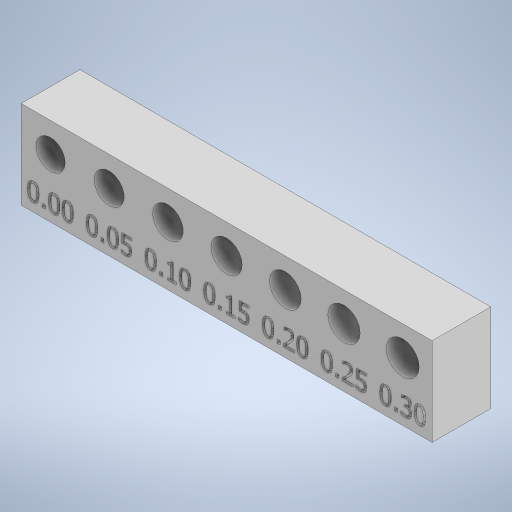
# Autodesk Inventor part: FIT TEST
Saved by Autodesk Inventor 2023 (Build 270158000, 158)
## iProperties
Created: 2023-05-17
Part Number: FIT TEST
Material: Generic
Document SubType Name: Modeling
Designer: Louis
Density: 1 g/cm^3
Appearance: Default
Author: Louis
Autodesk Inventor part; units mm, degrees
ref_plane "YZ Plane" through (0, 0, 0) normal (1, 0, 0) x (0, 1, 0)
ref_plane "XZ Plane" through (0, 0, 0) normal (0, 1, 0) x (-1, 0, 0)
ref_plane "XY Plane" through (0, 0, 0) normal (0, 0, 1) x (1, 0, 0)
sketch "Sketch1" plane through (0, 0, 0) normal (0, 0, 1) x (1, 0, 0)
  line L0 (0, 0) -> (10, 0)
  line L1 (10, 0) -> (10, 15)
  line L2 (10, 15) -> (0, 15)
  line L3 (0, 15) -> (0, 0)
  dimension "d0" = 10
  dimension "d1" = 15
  constraints: 8 end point, 2 parallel, 1 horizontal, 1 perpendicular
  measures "d0" distance of L1.end L2.end
  measures "d1" distance of L0.end L1.end
extrude "Extrusion1" add sketch "Sketch1" along normal blind 10
sketch "Sketch2" plane through (0, 0, 10) normal (0, 0, 1) x (1, 0, 0)
  line L0 (0, 15) -> (0, 0) projected
  line L1 (10, 15) -> (0, 15) projected
  point P0 (5, 10)
  dimension "d4" = 5
  dimension "d12" = 5
  measures "d4" distance from line of L0 point (5, 10)
  measures "d12" distance from line of L1 point (5, 10)
hole "Hole1" at (5, 10, 10) direction (0, 0, -1) diameter 5 end through all
pattern_linear "Rectangular Pattern1" count 7 spacing 10 along (1, 0, 0) of "Hole1", "Extrusion1"
sketch "Sketch3" plane through (0, 0, 10) normal (0, 0, 1) x (1, 0, 0)
  line L0 (0, 15) -> (0, 0) projected
  line L1 (0, 0) -> (10, 0)
  line L2 (10, 0) -> (10, 15)
  line L3 (10, 15) -> (0, 15)
  line L4 (0, 15) -> (0, 0)
  line L5 (10, 0) -> (20, 0)
  line L6 (20, 0) -> (20, 15)
  line L7 (20, 15) -> (10, 15)
  line L8 (10, 15) -> (10, 0)
  line L9 (20, 15) -> (30, 15)
  line L10 (30, 15) -> (30, 0)
  line L11 (30, 0) -> (20, 0)
  line L12 (20, 0) -> (20, 15)
  line L13 (30, 0) -> (40, 0)
  line L14 (40, 0) -> (40, 15)
  line L15 (40, 15) -> (30, 15)
  line L16 (30, 15) -> (30, 0)
  line L17 (40, 15) -> (40, 0)
  line L18 (0.9344, 4.587) -> (9.0656, 4.587) construction
  line L19 (9.0656, 4.587) -> (9.0656, 1.413) construction
  line L20 (9.0656, 1.413) -> (0.9344, 1.413) construction
  line L21 (0.9344, 1.413) -> (0.9344, 4.587) construction
  line L22 (10.9344, 4.587) -> (19.0656, 4.587) construction
  line L23 (19.0656, 4.587) -> (19.0656, 1.413) construction
  line L24 (19.0656, 1.413) -> (10.9344, 1.413) construction
  line L25 (10.9344, 1.413) -> (10.9344, 4.587) construction
  line L26 (20.9344, 4.587) -> (29.0656, 4.587) construction
  line L27 (29.0656, 4.587) -> (29.0656, 1.413) construction
  line L28 (29.0656, 1.413) -> (20.9344, 1.413) construction
  line L29 (20.9344, 1.413) -> (20.9344, 4.587) construction
  line L30 (30.9344, 4.587) -> (39.0656, 4.587) construction
  line L31 (39.0656, 4.587) -> (39.0656, 1.413) construction
  line L32 (39.0656, 1.413) -> (30.9344, 1.413) construction
  line L33 (30.9344, 1.413) -> (30.9344, 4.587) construction
  line L34 (40.9344, 4.5882) -> (49.0656, 4.5882) construction
  line L35 (49.0656, 4.5882) -> (49.0656, 1.4118) construction
  line L36 (49.0656, 1.4118) -> (40.9344, 1.4118) construction
  line L37 (40.9344, 1.4118) -> (40.9344, 4.5882) construction
  line L38 (50.9344, 4.5882) -> (59.0656, 4.5882) construction
  line L39 (59.0656, 4.5882) -> (59.0656, 1.4118) construction
  line L40 (59.0656, 1.4118) -> (50.9344, 1.4118) construction
  line L41 (50.9344, 1.4118) -> (50.9344, 4.5882) construction
  line L42 (60.9344, 4.5882) -> (69.0656, 4.5882) construction
  line L43 (69.0656, 4.5882) -> (69.0656, 1.4118) construction
  line L44 (69.0656, 1.4118) -> (60.9344, 1.4118) construction
  line L45 (60.9344, 1.4118) -> (60.9344, 4.5882) construction
  line L46 (0, 0) -> (70, 0) projected
  line L47 (40, 15) -> (50, 15)
  line L48 (50, 15) -> (50, 0)
  line L49 (50, 0) -> (40, 0)
  line L50 (40, 0) -> (40, 15)
  line L51 (0, 0) -> (70, 0) projected
  line L52 (50, 15) -> (60, 15)
  line L53 (60, 15) -> (60, 0)
  line L54 (60, 0) -> (50, 0)
  line L55 (50, 0) -> (50, 15)
  line L56 (60, 15) -> (70, 15)
  line L57 (70, 15) -> (70, 0)
  line L58 (70, 0) -> (60, 0)
  line L59 (60, 0) -> (60, 15)
  line L60 (70, 0) -> (70, 15) projected
  line L61 (70, 15) -> (0, 15) projected
  line L62 (0, 15) -> (0, 0) projected
  line L63 (0, 3) -> (70, 3)
  spline S0 degree 2 poles (3.0536, 3.0012) (3.0536, 2.1812) (2.5769, 1.413) (2.0804, 1.413) knots 0 0 0 1 2 2 2
  spline S1 degree 2 poles (2.0804, 1.413) (1.5766, 1.413) (1.1048, 2.196) (1.1048, 2.9988) knots 0 0 0 1 2 2 2
  spline S2 degree 2 poles (1.1048, 2.9988) (1.1048, 3.8238) (1.5815, 4.587) (2.0804, 4.587) knots 0 0 0 1 2 2 2
  spline S3 degree 2 poles (2.0804, 4.587) (2.5819, 4.587) (3.0536, 3.7966) (3.0536, 3.0012) knots 0 0 0 1 2 2 2
  spline S4 degree 2 poles (2.53, 2.0725) (2.5893, 2.2232) (2.6387, 2.6875) (2.6387, 3.0012) knots 0 0 0 1 2 2 2
  spline S5 degree 2 poles (2.6387, 3.0012) (2.6387, 3.3149) (2.5893, 3.7768) (2.5275, 3.9324) knots 0 0 0 1 2 2 2
  spline S6 degree 2 poles (2.5275, 3.9324) (2.4658, 4.088) (2.2509, 4.2486) (2.0804, 4.2486) knots 0 0 0 1 2 2 2
  spline S7 degree 2 poles (2.0804, 4.2486) (1.91, 4.2486) (1.6902, 4.088) (1.626, 3.9275) knots 0 0 0 1 2 2 2
  spline S8 degree 2 poles (1.626, 3.9275) (1.5642, 3.7719) (1.5197, 3.2976) (1.5197, 2.9988) knots 0 0 0 1 2 2 2
  spline S9 degree 2 poles (1.5197, 2.9988) (1.5197, 2.6777) (1.5593, 2.2479) (1.6235, 2.0799) knots 0 0 0 1 2 2 2
  spline S10 degree 2 poles (1.6235, 2.0799) (1.6828, 1.9218) (1.9026, 1.7514) (2.0804, 1.7514) knots 0 0 0 1 2 2 2
  spline S11 degree 2 poles (2.0804, 1.7514) (2.2484, 1.7514) (2.4682, 1.912) (2.53, 2.0725) knots 0 0 0 1 2 2 2
  line L64 (4.0984, 1.4772) -> (3.6094, 1.4772)
  line L65 (3.6094, 1.4772) -> (3.6094, 2.0602)
  line L66 (3.6094, 2.0602) -> (4.0984, 2.0602)
  line L67 (4.0984, 2.0602) -> (4.0984, 1.4772)
  spline S12 degree 2 poles (6.6105, 3.0012) (6.6105, 2.1812) (6.1337, 1.413) (5.6373, 1.413) knots 0 0 0 1 2 2 2
  spline S13 degree 2 poles (5.6373, 1.413) (5.1334, 1.413) (4.6616, 2.196) (4.6616, 2.9988) knots 0 0 0 1 2 2 2
  spline S14 degree 2 poles (4.6616, 2.9988) (4.6616, 3.8238) (5.1383, 4.587) (5.6373, 4.587) knots 0 0 0 1 2 2 2
  spline S15 degree 2 poles (5.6373, 4.587) (6.1387, 4.587) (6.6105, 3.7966) (6.6105, 3.0012) knots 0 0 0 1 2 2 2
  spline S16 degree 2 poles (6.0868, 2.0725) (6.1461, 2.2232) (6.1955, 2.6875) (6.1955, 3.0012) knots 0 0 0 1 2 2 2
  spline S17 degree 2 poles (6.1955, 3.0012) (6.1955, 3.3149) (6.1461, 3.7768) (6.0843, 3.9324) knots 0 0 0 1 2 2 2
  spline S18 degree 2 poles (6.0843, 3.9324) (6.0226, 4.088) (5.8077, 4.2486) (5.6373, 4.2486) knots 0 0 0 1 2 2 2
  spline S19 degree 2 poles (5.6373, 4.2486) (5.4668, 4.2486) (5.247, 4.088) (5.1828, 3.9275) knots 0 0 0 1 2 2 2
  spline S20 degree 2 poles (5.1828, 3.9275) (5.121, 3.7719) (5.0766, 3.2976) (5.0766, 2.9988) knots 0 0 0 1 2 2 2
  spline S21 degree 2 poles (5.0766, 2.9988) (5.0766, 2.6777) (5.1161, 2.2479) (5.1803, 2.0799) knots 0 0 0 1 2 2 2
  spline S22 degree 2 poles (5.1803, 2.0799) (5.2396, 1.9218) (5.4594, 1.7514) (5.6373, 1.7514) knots 0 0 0 1 2 2 2
  spline S23 degree 2 poles (5.6373, 1.7514) (5.8052, 1.7514) (6.0251, 1.912) (6.0868, 2.0725) knots 0 0 0 1 2 2 2
  spline S24 degree 2 poles (8.8977, 3.0012) (8.8977, 2.1812) (8.421, 1.413) (7.9245, 1.413) knots 0 0 0 1 2 2 2
  spline S25 degree 2 poles (7.9245, 1.413) (7.4206, 1.413) (6.9488, 2.196) (6.9488, 2.9988) knots 0 0 0 1 2 2 2
  spline S26 degree 2 poles (6.9488, 2.9988) (6.9488, 3.8238) (7.4256, 4.587) (7.9245, 4.587) knots 0 0 0 1 2 2 2
  spline S27 degree 2 poles (7.9245, 4.587) (8.4259, 4.587) (8.8977, 3.7966) (8.8977, 3.0012) knots 0 0 0 1 2 2 2
  spline S28 degree 2 poles (8.374, 2.0725) (8.4333, 2.2232) (8.4827, 2.6875) (8.4827, 3.0012) knots 0 0 0 1 2 2 2
  spline S29 degree 2 poles (8.4827, 3.0012) (8.4827, 3.3149) (8.4333, 3.7768) (8.3716, 3.9324) knots 0 0 0 1 2 2 2
  spline S30 degree 2 poles (8.3716, 3.9324) (8.3098, 4.088) (8.0949, 4.2486) (7.9245, 4.2486) knots 0 0 0 1 2 2 2
  spline S31 degree 2 poles (7.9245, 4.2486) (7.7541, 4.2486) (7.5342, 4.088) (7.47, 3.9275) knots 0 0 0 1 2 2 2
  spline S32 degree 2 poles (7.47, 3.9275) (7.4083, 3.7719) (7.3638, 3.2976) (7.3638, 2.9988) knots 0 0 0 1 2 2 2
  spline S33 degree 2 poles (7.3638, 2.9988) (7.3638, 2.6777) (7.4033, 2.2479) (7.4675, 2.0799) knots 0 0 0 1 2 2 2
  spline S34 degree 2 poles (7.4675, 2.0799) (7.5268, 1.9218) (7.7467, 1.7514) (7.9245, 1.7514) knots 0 0 0 1 2 2 2
  spline S35 degree 2 poles (7.9245, 1.7514) (8.0925, 1.7514) (8.3123, 1.912) (8.374, 2.0725) knots 0 0 0 1 2 2 2
  spline S36 degree 2 poles (13.0536, 3.0012) (13.0536, 2.1812) (12.5769, 1.413) (12.0804, 1.413) knots 0 0 0 1 2 2 2
  spline S37 degree 2 poles (12.0804, 1.413) (11.5766, 1.413) (11.1048, 2.196) (11.1048, 2.9988) knots 0 0 0 1 2 2 2
  spline S38 degree 2 poles (11.1048, 2.9988) (11.1048, 3.8238) (11.5815, 4.587) (12.0804, 4.587) knots 0 0 0 1 2 2 2
  spline S39 degree 2 poles (12.0804, 4.587) (12.5819, 4.587) (13.0536, 3.7966) (13.0536, 3.0012) knots 0 0 0 1 2 2 2
  spline S40 degree 2 poles (12.53, 2.0725) (12.5893, 2.2232) (12.6387, 2.6875) (12.6387, 3.0012) knots 0 0 0 1 2 2 2
  spline S41 degree 2 poles (12.6387, 3.0012) (12.6387, 3.3149) (12.5893, 3.7768) (12.5275, 3.9324) knots 0 0 0 1 2 2 2
  spline S42 degree 2 poles (12.5275, 3.9324) (12.4658, 4.088) (12.2509, 4.2486) (12.0804, 4.2486) knots 0 0 0 1 2 2 2
  spline S43 degree 2 poles (12.0804, 4.2486) (11.91, 4.2486) (11.6902, 4.088) (11.626, 3.9275) knots 0 0 0 1 2 2 2
  spline S44 degree 2 poles (11.626, 3.9275) (11.5642, 3.7719) (11.5197, 3.2976) (11.5197, 2.9988) knots 0 0 0 1 2 2 2
  spline S45 degree 2 poles (11.5197, 2.9988) (11.5197, 2.6777) (11.5593, 2.2479) (11.6235, 2.0799) knots 0 0 0 1 2 2 2
  spline S46 degree 2 poles (11.6235, 2.0799) (11.6828, 1.9218) (11.9026, 1.7514) (12.0804, 1.7514) knots 0 0 0 1 2 2 2
  spline S47 degree 2 poles (12.0804, 1.7514) (12.2484, 1.7514) (12.4682, 1.912) (12.53, 2.0725) knots 0 0 0 1 2 2 2
  line L68 (14.0984, 1.4772) -> (13.6094, 1.4772)
  line L69 (13.6094, 1.4772) -> (13.6094, 2.0602)
  line L70 (13.6094, 2.0602) -> (14.0984, 2.0602)
  line L71 (14.0984, 2.0602) -> (14.0984, 1.4772)
  spline S48 degree 2 poles (16.6105, 3.0012) (16.6105, 2.1812) (16.1337, 1.413) (15.6373, 1.413) knots 0 0 0 1 2 2 2
  spline S49 degree 2 poles (15.6373, 1.413) (15.1334, 1.413) (14.6616, 2.196) (14.6616, 2.9988) knots 0 0 0 1 2 2 2
  spline S50 degree 2 poles (14.6616, 2.9988) (14.6616, 3.8238) (15.1383, 4.587) (15.6373, 4.587) knots 0 0 0 1 2 2 2
  spline S51 degree 2 poles (15.6373, 4.587) (16.1387, 4.587) (16.6105, 3.7966) (16.6105, 3.0012) knots 0 0 0 1 2 2 2
  spline S52 degree 2 poles (16.0868, 2.0725) (16.1461, 2.2232) (16.1955, 2.6875) (16.1955, 3.0012) knots 0 0 0 1 2 2 2
  spline S53 degree 2 poles (16.1955, 3.0012) (16.1955, 3.3149) (16.1461, 3.7768) (16.0843, 3.9324) knots 0 0 0 1 2 2 2
  spline S54 degree 2 poles (16.0843, 3.9324) (16.0226, 4.088) (15.8077, 4.2486) (15.6373, 4.2486) knots 0 0 0 1 2 2 2
  spline S55 degree 2 poles (15.6373, 4.2486) (15.4668, 4.2486) (15.247, 4.088) (15.1828, 3.9275) knots 0 0 0 1 2 2 2
  spline S56 degree 2 poles (15.1828, 3.9275) (15.121, 3.7719) (15.0766, 3.2976) (15.0766, 2.9988) knots 0 0 0 1 2 2 2
  spline S57 degree 2 poles (15.0766, 2.9988) (15.0766, 2.6777) (15.1161, 2.2479) (15.1803, 2.0799) knots 0 0 0 1 2 2 2
  spline S58 degree 2 poles (15.1803, 2.0799) (15.2396, 1.9218) (15.4594, 1.7514) (15.6373, 1.7514) knots 0 0 0 1 2 2 2
  spline S59 degree 2 poles (15.6373, 1.7514) (15.8052, 1.7514) (16.0251, 1.912) (16.0868, 2.0725) knots 0 0 0 1 2 2 2
  spline S60 degree 2 poles (18.8483, 2.4455) (18.8483, 2.2256) (18.7075, 1.8502) (18.5791, 1.7119) knots 0 0 0 1 2 2 2
  spline S61 degree 2 poles (18.5791, 1.7119) (18.4506, 1.5736) (18.0678, 1.413) (17.8306, 1.413) knots 0 0 0 1 2 2 2
  spline S62 degree 2 poles (17.8306, 1.413) (17.6133, 1.413) (17.1884, 1.5093) (17.0328, 1.5859) knots 0 0 0 1 2 2 2
  line L72 (17.0328, 1.5859) -> (17.0328, 2.0182)
  line L73 (17.0328, 2.0182) -> (17.0625, 2.0182)
  spline S63 degree 2 poles (17.0625, 2.0182) (17.1094, 1.9836) (17.2848, 1.8947) (17.391, 1.8551) knots 0 0 0 1 2 2 2
  spline S64 degree 2 poles (17.391, 1.8551) (17.512, 1.8132) (17.7121, 1.7662) (17.838, 1.7662) knots 0 0 0 1 2 2 2
  spline S65 degree 2 poles (17.838, 1.7662) (17.9615, 1.7662) (18.1937, 1.8551) (18.2777, 1.9515) knots 0 0 0 1 2 2 2
  spline S66 degree 2 poles (18.2777, 1.9515) (18.3543, 2.0429) (18.4333, 2.2849) (18.4333, 2.448) knots 0 0 0 1 2 2 2
  spline S67 degree 2 poles (18.4333, 2.448) (18.4333, 2.611) (18.3444, 2.8185) (18.2604, 2.8876) knots 0 0 0 1 2 2 2
  spline S68 degree 2 poles (18.2604, 2.8876) (18.174, 2.9642) (17.9171, 3.0284) (17.7615, 3.0284) knots 0 0 0 1 2 2 2
  spline S69 degree 2 poles (17.7615, 3.0284) (17.5935, 3.0284) (17.2601, 2.9765) (17.1588, 2.9543) knots 0 0 0 1 2 2 2
  line L74 (17.1588, 2.9543) -> (17.1588, 4.5252)
  line L75 (17.1588, 4.5252) -> (18.831, 4.5252)
  line L76 (18.831, 4.5252) -> (18.831, 4.1671)
  line L77 (18.831, 4.1671) -> (17.5515, 4.1671)
  line L78 (17.5515, 4.1671) -> (17.5515, 3.3544)
  spline S70 degree 2 poles (17.5515, 3.3544) (17.6256, 3.3643) (17.7689, 3.3717) (17.8282, 3.3717) knots 0 0 0 1 2 2 2
  spline S71 degree 2 poles (17.8282, 3.3717) (18.0628, 3.3717) (18.3864, 3.2952) (18.5346, 3.1815) knots 0 0 0 1 2 2 2
  spline S72 degree 2 poles (18.5346, 3.1815) (18.6853, 3.0679) (18.8483, 2.7221) (18.8483, 2.4455) knots 0 0 0 1 2 2 2
  spline S73 degree 2 poles (23.0536, 3.0012) (23.0536, 2.1812) (22.5769, 1.413) (22.0804, 1.413) knots 0 0 0 1 2 2 2
  spline S74 degree 2 poles (22.0804, 1.413) (21.5766, 1.413) (21.1048, 2.196) (21.1048, 2.9988) knots 0 0 0 1 2 2 2
  spline S75 degree 2 poles (21.1048, 2.9988) (21.1048, 3.8238) (21.5815, 4.587) (22.0804, 4.587) knots 0 0 0 1 2 2 2
  spline S76 degree 2 poles (22.0804, 4.587) (22.5819, 4.587) (23.0536, 3.7966) (23.0536, 3.0012) knots 0 0 0 1 2 2 2
  spline S77 degree 2 poles (22.53, 2.0725) (22.5893, 2.2232) (22.6387, 2.6875) (22.6387, 3.0012) knots 0 0 0 1 2 2 2
  spline S78 degree 2 poles (22.6387, 3.0012) (22.6387, 3.3149) (22.5893, 3.7768) (22.5275, 3.9324) knots 0 0 0 1 2 2 2
  spline S79 degree 2 poles (22.5275, 3.9324) (22.4658, 4.088) (22.2509, 4.2486) (22.0804, 4.2486) knots 0 0 0 1 2 2 2
  spline S80 degree 2 poles (22.0804, 4.2486) (21.91, 4.2486) (21.6902, 4.088) (21.626, 3.9275) knots 0 0 0 1 2 2 2
  spline S81 degree 2 poles (21.626, 3.9275) (21.5642, 3.7719) (21.5197, 3.2976) (21.5197, 2.9988) knots 0 0 0 1 2 2 2
  spline S82 degree 2 poles (21.5197, 2.9988) (21.5197, 2.6777) (21.5593, 2.2479) (21.6235, 2.0799) knots 0 0 0 1 2 2 2
  spline S83 degree 2 poles (21.6235, 2.0799) (21.6828, 1.9218) (21.9026, 1.7514) (22.0804, 1.7514) knots 0 0 0 1 2 2 2
  spline S84 degree 2 poles (22.0804, 1.7514) (22.2484, 1.7514) (22.4682, 1.912) (22.53, 2.0725) knots 0 0 0 1 2 2 2
  line L79 (24.0984, 1.4772) -> (23.6094, 1.4772)
  line L80 (23.6094, 1.4772) -> (23.6094, 2.0602)
  line L81 (23.6094, 2.0602) -> (24.0984, 2.0602)
  line L82 (24.0984, 2.0602) -> (24.0984, 1.4772)
  line L83 (26.44, 1.4772) -> (24.9531, 1.4772)
  line L84 (24.9531, 1.4772) -> (24.9531, 1.7885)
  line L85 (24.9531, 1.7885) -> (25.5064, 1.7885)
  line L86 (25.5064, 1.7885) -> (25.5064, 3.8312)
  line L87 (25.5064, 3.8312) -> (24.9531, 3.8312)
  line L88 (24.9531, 3.8312) -> (24.9531, 4.1103)
  spline S85 degree 2 poles (24.9531, 4.1103) (25.2668, 4.1103) (25.5632, 4.2881) (25.5829, 4.5351) knots 0 0 0 1 2 2 2
  line L89 (25.5829, 4.5351) -> (25.8991, 4.5351)
  line L90 (25.8991, 4.5351) -> (25.8991, 1.7885)
  line L91 (25.8991, 1.7885) -> (26.44, 1.7885)
  line L92 (26.44, 1.7885) -> (26.44, 1.4772)
  spline S86 degree 2 poles (28.8977, 3.0012) (28.8977, 2.1812) (28.421, 1.413) (27.9245, 1.413) knots 0 0 0 1 2 2 2
  spline S87 degree 2 poles (27.9245, 1.413) (27.4206, 1.413) (26.9488, 2.196) (26.9488, 2.9988) knots 0 0 0 1 2 2 2
  spline S88 degree 2 poles (26.9488, 2.9988) (26.9488, 3.8238) (27.4256, 4.587) (27.9245, 4.587) knots 0 0 0 1 2 2 2
  spline S89 degree 2 poles (27.9245, 4.587) (28.4259, 4.587) (28.8977, 3.7966) (28.8977, 3.0012) knots 0 0 0 1 2 2 2
  spline S90 degree 2 poles (28.374, 2.0725) (28.4333, 2.2232) (28.4827, 2.6875) (28.4827, 3.0012) knots 0 0 0 1 2 2 2
  spline S91 degree 2 poles (28.4827, 3.0012) (28.4827, 3.3149) (28.4333, 3.7768) (28.3716, 3.9324) knots 0 0 0 1 2 2 2
  spline S92 degree 2 poles (28.3716, 3.9324) (28.3098, 4.088) (28.0949, 4.2486) (27.9245, 4.2486) knots 0 0 0 1 2 2 2
  spline S93 degree 2 poles (27.9245, 4.2486) (27.7541, 4.2486) (27.5342, 4.088) (27.47, 3.9275) knots 0 0 0 1 2 2 2
  spline S94 degree 2 poles (27.47, 3.9275) (27.4083, 3.7719) (27.3638, 3.2976) (27.3638, 2.9988) knots 0 0 0 1 2 2 2
  spline S95 degree 2 poles (27.3638, 2.9988) (27.3638, 2.6777) (27.4033, 2.2479) (27.4675, 2.0799) knots 0 0 0 1 2 2 2
  spline S96 degree 2 poles (27.4675, 2.0799) (27.5268, 1.9218) (27.7467, 1.7514) (27.9245, 1.7514) knots 0 0 0 1 2 2 2
  spline S97 degree 2 poles (27.9245, 1.7514) (28.0925, 1.7514) (28.3123, 1.912) (28.374, 2.0725) knots 0 0 0 1 2 2 2
  spline S98 degree 2 poles (33.0536, 3.0012) (33.0536, 2.1812) (32.5769, 1.413) (32.0804, 1.413) knots 0 0 0 1 2 2 2
  spline S99 degree 2 poles (32.0804, 1.413) (31.5766, 1.413) (31.1048, 2.196) (31.1048, 2.9988) knots 0 0 0 1 2 2 2
  spline S100 degree 2 poles (31.1048, 2.9988) (31.1048, 3.8238) (31.5815, 4.587) (32.0804, 4.587) knots 0 0 0 1 2 2 2
  spline S101 degree 2 poles (32.0804, 4.587) (32.5819, 4.587) (33.0536, 3.7966) (33.0536, 3.0012) knots 0 0 0 1 2 2 2
  spline S102 degree 2 poles (32.53, 2.0725) (32.5893, 2.2232) (32.6387, 2.6875) (32.6387, 3.0012) knots 0 0 0 1 2 2 2
  spline S103 degree 2 poles (32.6387, 3.0012) (32.6387, 3.3149) (32.5893, 3.7768) (32.5275, 3.9324) knots 0 0 0 1 2 2 2
  spline S104 degree 2 poles (32.5275, 3.9324) (32.4658, 4.088) (32.2509, 4.2486) (32.0804, 4.2486) knots 0 0 0 1 2 2 2
  spline S105 degree 2 poles (32.0804, 4.2486) (31.91, 4.2486) (31.6902, 4.088) (31.626, 3.9275) knots 0 0 0 1 2 2 2
  spline S106 degree 2 poles (31.626, 3.9275) (31.5642, 3.7719) (31.5197, 3.2976) (31.5197, 2.9988) knots 0 0 0 1 2 2 2
  spline S107 degree 2 poles (31.5197, 2.9988) (31.5197, 2.6777) (31.5593, 2.2479) (31.6235, 2.0799) knots 0 0 0 1 2 2 2
  spline S108 degree 2 poles (31.6235, 2.0799) (31.6828, 1.9218) (31.9026, 1.7514) (32.0804, 1.7514) knots 0 0 0 1 2 2 2
  spline S109 degree 2 poles (32.0804, 1.7514) (32.2484, 1.7514) (32.4682, 1.912) (32.53, 2.0725) knots 0 0 0 1 2 2 2
  line L93 (34.0984, 1.4772) -> (33.6094, 1.4772)
  line L94 (33.6094, 1.4772) -> (33.6094, 2.0602)
  line L95 (33.6094, 2.0602) -> (34.0984, 2.0602)
  line L96 (34.0984, 2.0602) -> (34.0984, 1.4772)
  line L97 (36.44, 1.4772) -> (34.9531, 1.4772)
  line L98 (34.9531, 1.4772) -> (34.9531, 1.7885)
  line L99 (34.9531, 1.7885) -> (35.5064, 1.7885)
  line L100 (35.5064, 1.7885) -> (35.5064, 3.8312)
  line L101 (35.5064, 3.8312) -> (34.9531, 3.8312)
  line L102 (34.9531, 3.8312) -> (34.9531, 4.1103)
  spline S110 degree 2 poles (34.9531, 4.1103) (35.2668, 4.1103) (35.5632, 4.2881) (35.5829, 4.5351) knots 0 0 0 1 2 2 2
  line L103 (35.5829, 4.5351) -> (35.8991, 4.5351)
  line L104 (35.8991, 4.5351) -> (35.8991, 1.7885)
  line L105 (35.8991, 1.7885) -> (36.44, 1.7885)
  line L106 (36.44, 1.7885) -> (36.44, 1.4772)
  spline S111 degree 2 poles (38.8483, 2.4455) (38.8483, 2.2256) (38.7075, 1.8502) (38.5791, 1.7119) knots 0 0 0 1 2 2 2
  spline S112 degree 2 poles (38.5791, 1.7119) (38.4506, 1.5736) (38.0678, 1.413) (37.8306, 1.413) knots 0 0 0 1 2 2 2
  spline S113 degree 2 poles (37.8306, 1.413) (37.6133, 1.413) (37.1884, 1.5093) (37.0328, 1.5859) knots 0 0 0 1 2 2 2
  line L107 (37.0328, 1.5859) -> (37.0328, 2.0182)
  line L108 (37.0328, 2.0182) -> (37.0625, 2.0182)
  spline S114 degree 2 poles (37.0625, 2.0182) (37.1094, 1.9836) (37.2848, 1.8947) (37.391, 1.8551) knots 0 0 0 1 2 2 2
  spline S115 degree 2 poles (37.391, 1.8551) (37.512, 1.8132) (37.7121, 1.7662) (37.838, 1.7662) knots 0 0 0 1 2 2 2
  spline S116 degree 2 poles (37.838, 1.7662) (37.9615, 1.7662) (38.1937, 1.8551) (38.2777, 1.9515) knots 0 0 0 1 2 2 2
  spline S117 degree 2 poles (38.2777, 1.9515) (38.3543, 2.0429) (38.4333, 2.2849) (38.4333, 2.448) knots 0 0 0 1 2 2 2
  spline S118 degree 2 poles (38.4333, 2.448) (38.4333, 2.611) (38.3444, 2.8185) (38.2604, 2.8876) knots 0 0 0 1 2 2 2
  spline S119 degree 2 poles (38.2604, 2.8876) (38.174, 2.9642) (37.9171, 3.0284) (37.7615, 3.0284) knots 0 0 0 1 2 2 2
  spline S120 degree 2 poles (37.7615, 3.0284) (37.5935, 3.0284) (37.2601, 2.9765) (37.1588, 2.9543) knots 0 0 0 1 2 2 2
  line L109 (37.1588, 2.9543) -> (37.1588, 4.5252)
  line L110 (37.1588, 4.5252) -> (38.831, 4.5252)
  line L111 (38.831, 4.5252) -> (38.831, 4.1671)
  line L112 (38.831, 4.1671) -> (37.5515, 4.1671)
  line L113 (37.5515, 4.1671) -> (37.5515, 3.3544)
  spline S121 degree 2 poles (37.5515, 3.3544) (37.6256, 3.3643) (37.7689, 3.3717) (37.8282, 3.3717) knots 0 0 0 1 2 2 2
  spline S122 degree 2 poles (37.8282, 3.3717) (38.0628, 3.3717) (38.3864, 3.2952) (38.5346, 3.1815) knots 0 0 0 1 2 2 2
  spline S123 degree 2 poles (38.5346, 3.1815) (38.6853, 3.0679) (38.8483, 2.7221) (38.8483, 2.4455) knots 0 0 0 1 2 2 2
  spline S124 degree 2 poles (43.0536, 3) (43.0536, 2.18) (42.5769, 1.4118) (42.0804, 1.4118) knots 0 0 0 1 2 2 2
  spline S125 degree 2 poles (42.0804, 1.4118) (41.5766, 1.4118) (41.1048, 2.1948) (41.1048, 2.9975) knots 0 0 0 1 2 2 2
  spline S126 degree 2 poles (41.1048, 2.9975) (41.1048, 3.8225) (41.5815, 4.5858) (42.0804, 4.5858) knots 0 0 0 1 2 2 2
  spline S127 degree 2 poles (42.0804, 4.5858) (42.5819, 4.5858) (43.0536, 3.7953) (43.0536, 3) knots 0 0 0 1 2 2 2
  spline S128 degree 2 poles (42.53, 2.0713) (42.5893, 2.2219) (42.6387, 2.6863) (42.6387, 3) knots 0 0 0 1 2 2 2
  spline S129 degree 2 poles (42.6387, 3) (42.6387, 3.3137) (42.5893, 3.7756) (42.5275, 3.9312) knots 0 0 0 1 2 2 2
  spline S130 degree 2 poles (42.5275, 3.9312) (42.4658, 4.0868) (42.2509, 4.2474) (42.0804, 4.2474) knots 0 0 0 1 2 2 2
  spline S131 degree 2 poles (42.0804, 4.2474) (41.91, 4.2474) (41.6902, 4.0868) (41.626, 3.9263) knots 0 0 0 1 2 2 2
  spline S132 degree 2 poles (41.626, 3.9263) (41.5642, 3.7706) (41.5197, 3.2964) (41.5197, 2.9975) knots 0 0 0 1 2 2 2
  spline S133 degree 2 poles (41.5197, 2.9975) (41.5197, 2.6764) (41.5593, 2.2466) (41.6235, 2.0787) knots 0 0 0 1 2 2 2
  spline S134 degree 2 poles (41.6235, 2.0787) (41.6828, 1.9206) (41.9026, 1.7502) (42.0804, 1.7502) knots 0 0 0 1 2 2 2
  spline S135 degree 2 poles (42.0804, 1.7502) (42.2484, 1.7502) (42.4682, 1.9107) (42.53, 2.0713) knots 0 0 0 1 2 2 2
  line L114 (44.0984, 1.476) -> (43.6094, 1.476)
  line L115 (43.6094, 1.476) -> (43.6094, 2.0589)
  line L116 (43.6094, 2.0589) -> (44.0984, 2.0589)
  line L117 (44.0984, 2.0589) -> (44.0984, 1.476)
  line L118 (46.5932, 1.476) -> (44.7135, 1.476)
  line L119 (44.7135, 1.476) -> (44.7135, 1.9083)
  spline S136 degree 2 poles (44.7135, 1.9083) (44.916, 2.0984) (45.2766, 2.4517) (45.4495, 2.6418) knots 0 0 0 1 2 2 2
  spline S137 degree 2 poles (45.4495, 2.6418) (45.7978, 3.0247) (46.0522, 3.4841) (46.0522, 3.7287) knots 0 0 0 1 2 2 2
  spline S138 degree 2 poles (46.0522, 3.7287) (46.0522, 3.8571) (45.9732, 4.0498) (45.9016, 4.1115) knots 0 0 0 1 2 2 2
  spline S139 degree 2 poles (45.9016, 4.1115) (45.8299, 4.1733) (45.6422, 4.235) (45.5286, 4.235) knots 0 0 0 1 2 2 2
  spline S140 degree 2 poles (45.5286, 4.235) (45.4199, 4.235) (45.1976, 4.1807) (45.0963, 4.1387) knots 0 0 0 1 2 2 2
  spline S141 degree 2 poles (45.0963, 4.1387) (45.0099, 4.1041) (44.8493, 4.0053) (44.7999, 3.9707) knots 0 0 0 1 2 2 2
  line L120 (44.7999, 3.9707) -> (44.7777, 3.9707)
  line L121 (44.7777, 3.9707) -> (44.7777, 4.4054)
  spline S142 degree 2 poles (44.7777, 4.4054) (44.9037, 4.4672) (45.3557, 4.5882) (45.5582, 4.5882) knots 0 0 0 1 2 2 2
  spline S143 degree 2 poles (45.5582, 4.5882) (45.9855, 4.5882) (46.4672, 4.1362) (46.4672, 3.7509) knots 0 0 0 1 2 2 2
  spline S144 degree 2 poles (46.4672, 3.7509) (46.4672, 3.5706) (46.3832, 3.2692) (46.3091, 3.1408) knots 0 0 0 1 2 2 2
  spline S145 degree 2 poles (46.3091, 3.1408) (46.235, 3.0074) (46.0201, 2.7456) (45.9016, 2.6196) knots 0 0 0 1 2 2 2
  spline S146 degree 2 poles (45.9016, 2.6196) (45.7089, 2.4097) (45.2371, 1.9601) (45.0963, 1.8292) knots 0 0 0 1 2 2 2
  line L122 (45.0963, 1.8292) -> (46.5932, 1.8292)
  line L123 (46.5932, 1.8292) -> (46.5932, 1.476)
  spline S147 degree 2 poles (48.8977, 3) (48.8977, 2.18) (48.421, 1.4118) (47.9245, 1.4118) knots 0 0 0 1 2 2 2
  spline S148 degree 2 poles (47.9245, 1.4118) (47.4206, 1.4118) (46.9488, 2.1948) (46.9488, 2.9975) knots 0 0 0 1 2 2 2
  spline S149 degree 2 poles (46.9488, 2.9975) (46.9488, 3.8225) (47.4256, 4.5858) (47.9245, 4.5858) knots 0 0 0 1 2 2 2
  spline S150 degree 2 poles (47.9245, 4.5858) (48.4259, 4.5858) (48.8977, 3.7953) (48.8977, 3) knots 0 0 0 1 2 2 2
  spline S151 degree 2 poles (48.374, 2.0713) (48.4333, 2.2219) (48.4827, 2.6863) (48.4827, 3) knots 0 0 0 1 2 2 2
  spline S152 degree 2 poles (48.4827, 3) (48.4827, 3.3137) (48.4333, 3.7756) (48.3716, 3.9312) knots 0 0 0 1 2 2 2
  spline S153 degree 2 poles (48.3716, 3.9312) (48.3098, 4.0868) (48.0949, 4.2474) (47.9245, 4.2474) knots 0 0 0 1 2 2 2
  spline S154 degree 2 poles (47.9245, 4.2474) (47.7541, 4.2474) (47.5342, 4.0868) (47.47, 3.9263) knots 0 0 0 1 2 2 2
  spline S155 degree 2 poles (47.47, 3.9263) (47.4083, 3.7706) (47.3638, 3.2964) (47.3638, 2.9975) knots 0 0 0 1 2 2 2
  spline S156 degree 2 poles (47.3638, 2.9975) (47.3638, 2.6764) (47.4033, 2.2466) (47.4675, 2.0787) knots 0 0 0 1 2 2 2
  spline S157 degree 2 poles (47.4675, 2.0787) (47.5268, 1.9206) (47.7467, 1.7502) (47.9245, 1.7502) knots 0 0 0 1 2 2 2
  spline S158 degree 2 poles (47.9245, 1.7502) (48.0925, 1.7502) (48.3123, 1.9107) (48.374, 2.0713) knots 0 0 0 1 2 2 2
  spline S159 degree 2 poles (53.0536, 3) (53.0536, 2.18) (52.5769, 1.4118) (52.0804, 1.4118) knots 0 0 0 1 2 2 2
  spline S160 degree 2 poles (52.0804, 1.4118) (51.5766, 1.4118) (51.1048, 2.1948) (51.1048, 2.9975) knots 0 0 0 1 2 2 2
  spline S161 degree 2 poles (51.1048, 2.9975) (51.1048, 3.8225) (51.5815, 4.5858) (52.0804, 4.5858) knots 0 0 0 1 2 2 2
  spline S162 degree 2 poles (52.0804, 4.5858) (52.5819, 4.5858) (53.0536, 3.7953) (53.0536, 3) knots 0 0 0 1 2 2 2
  spline S163 degree 2 poles (52.53, 2.0713) (52.5893, 2.2219) (52.6387, 2.6863) (52.6387, 3) knots 0 0 0 1 2 2 2
  spline S164 degree 2 poles (52.6387, 3) (52.6387, 3.3137) (52.5893, 3.7756) (52.5275, 3.9312) knots 0 0 0 1 2 2 2
  spline S165 degree 2 poles (52.5275, 3.9312) (52.4658, 4.0868) (52.2509, 4.2474) (52.0804, 4.2474) knots 0 0 0 1 2 2 2
  spline S166 degree 2 poles (52.0804, 4.2474) (51.91, 4.2474) (51.6902, 4.0868) (51.626, 3.9263) knots 0 0 0 1 2 2 2
  spline S167 degree 2 poles (51.626, 3.9263) (51.5642, 3.7706) (51.5197, 3.2964) (51.5197, 2.9975) knots 0 0 0 1 2 2 2
  spline S168 degree 2 poles (51.5197, 2.9975) (51.5197, 2.6764) (51.5593, 2.2466) (51.6235, 2.0787) knots 0 0 0 1 2 2 2
  spline S169 degree 2 poles (51.6235, 2.0787) (51.6828, 1.9206) (51.9026, 1.7502) (52.0804, 1.7502) knots 0 0 0 1 2 2 2
  spline S170 degree 2 poles (52.0804, 1.7502) (52.2484, 1.7502) (52.4682, 1.9107) (52.53, 2.0713) knots 0 0 0 1 2 2 2
  line L124 (54.0984, 1.476) -> (53.6094, 1.476)
  line L125 (53.6094, 1.476) -> (53.6094, 2.0589)
  line L126 (53.6094, 2.0589) -> (54.0984, 2.0589)
  line L127 (54.0984, 2.0589) -> (54.0984, 1.476)
  line L128 (56.5932, 1.476) -> (54.7135, 1.476)
  line L129 (54.7135, 1.476) -> (54.7135, 1.9083)
  spline S171 degree 2 poles (54.7135, 1.9083) (54.916, 2.0984) (55.2766, 2.4517) (55.4495, 2.6418) knots 0 0 0 1 2 2 2
  spline S172 degree 2 poles (55.4495, 2.6418) (55.7978, 3.0247) (56.0522, 3.4841) (56.0522, 3.7287) knots 0 0 0 1 2 2 2
  spline S173 degree 2 poles (56.0522, 3.7287) (56.0522, 3.8571) (55.9732, 4.0498) (55.9016, 4.1115) knots 0 0 0 1 2 2 2
  spline S174 degree 2 poles (55.9016, 4.1115) (55.8299, 4.1733) (55.6422, 4.235) (55.5286, 4.235) knots 0 0 0 1 2 2 2
  spline S175 degree 2 poles (55.5286, 4.235) (55.4199, 4.235) (55.1976, 4.1807) (55.0963, 4.1387) knots 0 0 0 1 2 2 2
  spline S176 degree 2 poles (55.0963, 4.1387) (55.0099, 4.1041) (54.8493, 4.0053) (54.7999, 3.9707) knots 0 0 0 1 2 2 2
  line L130 (54.7999, 3.9707) -> (54.7777, 3.9707)
  line L131 (54.7777, 3.9707) -> (54.7777, 4.4054)
  spline S177 degree 2 poles (54.7777, 4.4054) (54.9037, 4.4672) (55.3557, 4.5882) (55.5582, 4.5882) knots 0 0 0 1 2 2 2
  spline S178 degree 2 poles (55.5582, 4.5882) (55.9855, 4.5882) (56.4672, 4.1362) (56.4672, 3.7509) knots 0 0 0 1 2 2 2
  spline S179 degree 2 poles (56.4672, 3.7509) (56.4672, 3.5706) (56.3832, 3.2692) (56.3091, 3.1408) knots 0 0 0 1 2 2 2
  spline S180 degree 2 poles (56.3091, 3.1408) (56.235, 3.0074) (56.0201, 2.7456) (55.9016, 2.6196) knots 0 0 0 1 2 2 2
  spline S181 degree 2 poles (55.9016, 2.6196) (55.7089, 2.4097) (55.2371, 1.9601) (55.0963, 1.8292) knots 0 0 0 1 2 2 2
  line L132 (55.0963, 1.8292) -> (56.5932, 1.8292)
  line L133 (56.5932, 1.8292) -> (56.5932, 1.476)
  spline S182 degree 2 poles (58.8483, 2.4442) (58.8483, 2.2244) (58.7075, 1.849) (58.5791, 1.7107) knots 0 0 0 1 2 2 2
  spline S183 degree 2 poles (58.5791, 1.7107) (58.4506, 1.5723) (58.0678, 1.4118) (57.8306, 1.4118) knots 0 0 0 1 2 2 2
  spline S184 degree 2 poles (57.8306, 1.4118) (57.6133, 1.4118) (57.1884, 1.5081) (57.0328, 1.5847) knots 0 0 0 1 2 2 2
  line L134 (57.0328, 1.5847) -> (57.0328, 2.0169)
  line L135 (57.0328, 2.0169) -> (57.0625, 2.0169)
  spline S185 degree 2 poles (57.0625, 2.0169) (57.1094, 1.9824) (57.2848, 1.8934) (57.391, 1.8539) knots 0 0 0 1 2 2 2
  spline S186 degree 2 poles (57.391, 1.8539) (57.512, 1.8119) (57.7121, 1.765) (57.838, 1.765) knots 0 0 0 1 2 2 2
  spline S187 degree 2 poles (57.838, 1.765) (57.9615, 1.765) (58.1937, 1.8539) (58.2777, 1.9502) knots 0 0 0 1 2 2 2
  spline S188 degree 2 poles (58.2777, 1.9502) (58.3543, 2.0416) (58.4333, 2.2837) (58.4333, 2.4467) knots 0 0 0 1 2 2 2
  spline S189 degree 2 poles (58.4333, 2.4467) (58.4333, 2.6097) (58.3444, 2.8172) (58.2604, 2.8864) knots 0 0 0 1 2 2 2
  spline S190 degree 2 poles (58.2604, 2.8864) (58.174, 2.9629) (57.9171, 3.0272) (57.7615, 3.0272) knots 0 0 0 1 2 2 2
  spline S191 degree 2 poles (57.7615, 3.0272) (57.5935, 3.0272) (57.2601, 2.9753) (57.1588, 2.9531) knots 0 0 0 1 2 2 2
  line L136 (57.1588, 2.9531) -> (57.1588, 4.524)
  line L137 (57.1588, 4.524) -> (58.831, 4.524)
  line L138 (58.831, 4.524) -> (58.831, 4.1658)
  line L139 (58.831, 4.1658) -> (57.5515, 4.1658)
  line L140 (57.5515, 4.1658) -> (57.5515, 3.3532)
  spline S192 degree 2 poles (57.5515, 3.3532) (57.6256, 3.3631) (57.7689, 3.3705) (57.8282, 3.3705) knots 0 0 0 1 2 2 2
  spline S193 degree 2 poles (57.8282, 3.3705) (58.0628, 3.3705) (58.3864, 3.2939) (58.5346, 3.1803) knots 0 0 0 1 2 2 2
  spline S194 degree 2 poles (58.5346, 3.1803) (58.6853, 3.0667) (58.8483, 2.7209) (58.8483, 2.4442) knots 0 0 0 1 2 2 2
  spline S195 degree 2 poles (63.0536, 3) (63.0536, 2.18) (62.5769, 1.4118) (62.0804, 1.4118) knots 0 0 0 1 2 2 2
  spline S196 degree 2 poles (62.0804, 1.4118) (61.5766, 1.4118) (61.1048, 2.1948) (61.1048, 2.9975) knots 0 0 0 1 2 2 2
  spline S197 degree 2 poles (61.1048, 2.9975) (61.1048, 3.8225) (61.5815, 4.5858) (62.0804, 4.5858) knots 0 0 0 1 2 2 2
  spline S198 degree 2 poles (62.0804, 4.5858) (62.5819, 4.5858) (63.0536, 3.7953) (63.0536, 3) knots 0 0 0 1 2 2 2
  spline S199 degree 2 poles (62.53, 2.0713) (62.5893, 2.2219) (62.6387, 2.6863) (62.6387, 3) knots 0 0 0 1 2 2 2
  spline S200 degree 2 poles (62.6387, 3) (62.6387, 3.3137) (62.5893, 3.7756) (62.5275, 3.9312) knots 0 0 0 1 2 2 2
  spline S201 degree 2 poles (62.5275, 3.9312) (62.4658, 4.0868) (62.2509, 4.2474) (62.0804, 4.2474) knots 0 0 0 1 2 2 2
  spline S202 degree 2 poles (62.0804, 4.2474) (61.91, 4.2474) (61.6902, 4.0868) (61.626, 3.9263) knots 0 0 0 1 2 2 2
  spline S203 degree 2 poles (61.626, 3.9263) (61.5642, 3.7706) (61.5197, 3.2964) (61.5197, 2.9975) knots 0 0 0 1 2 2 2
  spline S204 degree 2 poles (61.5197, 2.9975) (61.5197, 2.6764) (61.5593, 2.2466) (61.6235, 2.0787) knots 0 0 0 1 2 2 2
  spline S205 degree 2 poles (61.6235, 2.0787) (61.6828, 1.9206) (61.9026, 1.7502) (62.0804, 1.7502) knots 0 0 0 1 2 2 2
  spline S206 degree 2 poles (62.0804, 1.7502) (62.2484, 1.7502) (62.4682, 1.9107) (62.53, 2.0713) knots 0 0 0 1 2 2 2
  line L141 (64.0984, 1.476) -> (63.6094, 1.476)
  line L142 (63.6094, 1.476) -> (63.6094, 2.0589)
  line L143 (63.6094, 2.0589) -> (64.0984, 2.0589)
  line L144 (64.0984, 2.0589) -> (64.0984, 1.476)
  spline S207 degree 2 poles (65.536, 4.235) (65.4248, 4.235) (65.205, 4.1807) (65.0988, 4.1387) knots 0 0 0 1 2 2 2
  spline S208 degree 2 poles (65.0988, 4.1387) (65, 4.0967) (64.8543, 4.0078) (64.7975, 3.9682) knots 0 0 0 1 2 2 2
  line L145 (64.7975, 3.9682) -> (64.7728, 3.9682)
  line L146 (64.7728, 3.9682) -> (64.7728, 4.4005)
  spline S209 degree 2 poles (64.7728, 4.4005) (64.9061, 4.4721) (65.3631, 4.5882) (65.5681, 4.5882) knots 0 0 0 1 2 2 2
  spline S210 degree 2 poles (65.5681, 4.5882) (65.7756, 4.5882) (66.0843, 4.5042) (66.2103, 4.4153) knots 0 0 0 1 2 2 2
  spline S211 degree 2 poles (66.2103, 4.4153) (66.3437, 4.319) (66.482, 4.0399) (66.482, 3.8522) knots 0 0 0 1 2 2 2
  spline S212 degree 2 poles (66.482, 3.8522) (66.482, 3.6002) (66.151, 3.2198) (65.9188, 3.1704) knots 0 0 0 1 2 2 2
  line L147 (65.9188, 3.1704) -> (65.9188, 3.1408)
  spline S213 degree 2 poles (65.9188, 3.1408) (66.0152, 3.121) (66.235, 3.0321) (66.3289, 2.9432) knots 0 0 0 1 2 2 2
  spline S214 degree 2 poles (66.3289, 2.9432) (66.4227, 2.8567) (66.5413, 2.5801) (66.5413, 2.38) knots 0 0 0 1 2 2 2
  spline S215 degree 2 poles (66.5413, 2.38) (66.5413, 2.175) (66.4005, 1.8267) (66.2721, 1.6934) knots 0 0 0 1 2 2 2
  spline S216 degree 2 poles (66.2721, 1.6934) (66.1387, 1.555) (65.7608, 1.4118) (65.5212, 1.4118) knots 0 0 0 1 2 2 2
  spline S217 degree 2 poles (65.5212, 1.4118) (65.2915, 1.4118) (64.8419, 1.5229) (64.6888, 1.5995) knots 0 0 0 1 2 2 2
  line L148 (64.6888, 1.5995) -> (64.6888, 2.0318)
  line L149 (64.6888, 2.0318) -> (64.7184, 2.0318)
  spline S218 degree 2 poles (64.7184, 2.0318) (64.8469, 1.9379) (65.2816, 1.765) (65.4965, 1.765) knots 0 0 0 1 2 2 2
  spline S219 degree 2 poles (65.4965, 1.765) (65.6224, 1.765) (65.8744, 1.844) (65.9584, 1.9354) knots 0 0 0 1 2 2 2
  spline S220 degree 2 poles (65.9584, 1.9354) (66.0399, 2.0268) (66.1263, 2.2442) (66.1263, 2.4097) knots 0 0 0 1 2 2 2
  spline S221 degree 2 poles (66.1263, 2.4097) (66.1263, 2.5752) (66.03, 2.79) (65.9435, 2.8518) knots 0 0 0 1 2 2 2
  spline S222 degree 2 poles (65.9435, 2.8518) (65.8571, 2.9135) (65.6224, 2.9605) (65.4841, 2.9605) knots 0 0 0 1 2 2 2
  line L150 (65.4841, 2.9605) -> (65.3112, 2.9605)
  line L151 (65.3112, 2.9605) -> (65.3112, 3.2989)
  line L152 (65.3112, 3.2989) -> (65.4471, 3.2989)
  spline S223 degree 2 poles (65.4471, 3.2989) (65.7212, 3.2989) (66.067, 3.5607) (66.067, 3.8102) knots 0 0 0 1 2 2 2
  spline S224 degree 2 poles (66.067, 3.8102) (66.067, 3.9263) (65.9781, 4.0917) (65.9065, 4.1411) knots 0 0 0 1 2 2 2
  spline S225 degree 2 poles (65.9065, 4.1411) (65.8299, 4.193) (65.6422, 4.235) (65.536, 4.235) knots 0 0 0 1 2 2 2
  spline S226 degree 2 poles (68.8977, 3) (68.8977, 2.18) (68.421, 1.4118) (67.9245, 1.4118) knots 0 0 0 1 2 2 2
  spline S227 degree 2 poles (67.9245, 1.4118) (67.4206, 1.4118) (66.9488, 2.1948) (66.9488, 2.9975) knots 0 0 0 1 2 2 2
  spline S228 degree 2 poles (66.9488, 2.9975) (66.9488, 3.8225) (67.4256, 4.5858) (67.9245, 4.5858) knots 0 0 0 1 2 2 2
  spline S229 degree 2 poles (67.9245, 4.5858) (68.4259, 4.5858) (68.8977, 3.7953) (68.8977, 3) knots 0 0 0 1 2 2 2
  spline S230 degree 2 poles (68.374, 2.0713) (68.4333, 2.2219) (68.4827, 2.6863) (68.4827, 3) knots 0 0 0 1 2 2 2
  spline S231 degree 2 poles (68.4827, 3) (68.4827, 3.3137) (68.4333, 3.7756) (68.3716, 3.9312) knots 0 0 0 1 2 2 2
  spline S232 degree 2 poles (68.3716, 3.9312) (68.3098, 4.0868) (68.0949, 4.2474) (67.9245, 4.2474) knots 0 0 0 1 2 2 2
  spline S233 degree 2 poles (67.9245, 4.2474) (67.7541, 4.2474) (67.5342, 4.0868) (67.47, 3.9263) knots 0 0 0 1 2 2 2
  spline S234 degree 2 poles (67.47, 3.9263) (67.4083, 3.7706) (67.3638, 3.2964) (67.3638, 2.9975) knots 0 0 0 1 2 2 2
  spline S235 degree 2 poles (67.3638, 2.9975) (67.3638, 2.6764) (67.4033, 2.2466) (67.4675, 2.0787) knots 0 0 0 1 2 2 2
  spline S236 degree 2 poles (67.4675, 2.0787) (67.5268, 1.9206) (67.7467, 1.7502) (67.9245, 1.7502) knots 0 0 0 1 2 2 2
  spline S237 degree 2 poles (67.9245, 1.7502) (68.0925, 1.7502) (68.3123, 1.9107) (68.374, 2.0713) knots 0 0 0 1 2 2 2
  point P0 (5, 4.587)
  point P1 (5, 15)
  point P2 (0.9344, 3)
  point P3 (15, 4.587)
  point P4 (15, 15)
  point P5 (10.9344, 3)
  point P6 (25, 4.587)
  point P7 (25, 15)
  point P8 (20.9344, 3)
  point P9 (35, 4.587)
  point P10 (35, 15)
  point P11 (30.9344, 3)
  point P12 (45, 4.5882)
  point P13 (40.9344, 3)
  point P14 (55, 4.5882)
  point P15 (55, 15)
  point P16 (50.9344, 3)
  point P17 (65, 4.5882)
  point P18 (65, 15)
  point P19 (60.9344, 3)
  dimension "d16" = 10
  dimension "d17" = 10
  dimension "d18" = 10
  dimension "d19" = 10
  dimension "d22" = 10
  dimension "d23" = 10
  dimension "d25" = 3
  constraints: 60 end point, 19 midpoint, 14 parallel, 9 horizontal, 8 perpendicular, 6 vertical alignment, 4 point on line, 2 horizontal alignment, 17 other
  measures "d16" distance between parallel lines of L4 L2
  measures "d17" distance between parallel lines of L6 L8
  measures "d18" distance between parallel lines of L10 L6
  measures "d19" distance between parallel lines of L14 L10
  measures "d22" distance between parallel lines of L48 L14
  measures "d23" distance between parallel lines of L55 L53
  measures "d25" distance of the line from the sketch origin of L63
extrude "Extrusion2" cut sketch "Sketch3" against normal blind 0.5 contours S2 S3 L63 S5 S6 S7 S8 | L63 S9 S10 S11 S4 S0 S1 | S24 S25 L63 S33 S34 S35 S28 | L63 S29 S30 S31 S32 S26 S27 | S38 S39 L63 S41 S42 S43 S44 | L63 S45 S46 S47 S40 S36 S37 | S72 S60 S61 S62 L72 L73 S63 S64 S65 S66 S67 S68 L63 | L63 S68 S69 L74 L75 L76 L77 L78 S70 S71 S72 | S75 S76 L63 S78 S79 S80 S81 | L63 S82 S83 S84 S77 S73 S74 | S14 S15 L63 S17 S18 S19 S20 | L63 S21 S22 S23 S16 S12 S13 | S86 S87 L63 S95 S96 S97 S90 | L63 S91 S92 S93 S94 S88 S89 | S100 S101 L63 S103 S104 S105 S106 | L63 S107 S108 S109 S102 S98 S99 | S50 S51 L63 S53 S54 S55 S56 | L63 S57 S58 S59 S52 S48 S49 | S69 L74 L63 | S123 S111 S112 S113 L107 L108 S114 S115 S116 S117 S118 S119 L63 | L63 S119 S120 L109 L110 L111 L112 L113 S121 S122 S123 | S126 S127 L63 S129 S130 S131 S132 | L63 S132 S133 S134 S135 S128 S124 S125 S126 | L86 L87 L88 S85 L89 L90 L63 | L63 L90 L91 L92 L83 L84 L85 L86 | S147 S148 S149 L63 S155 S156 S157 S158 S151 | L63 S152 S153 S154 S155 S149 S150 | S161 S162 L63 S164 S165 S166 S167 | L63 S167 S168 S169 S170 S163 S159 S160 S161 | L100 L101 L102 S110 L103 L104 L63 | L63 L104 L105 L106 L97 L98 L99 L100 | S120 L109 L63 | S194 S182 S183 S184 L134 L135 S185 S186 S187 S188 S189 S190 L63 | L63 S190 S191 L136 L137 L138 L139 L140 S192 S193 S194 | S197 S198 L63 S200 S201 S202 S203 | L63 S203 S204 S205 S206 S199 S195 S196 S197 | S137 S138 S139 S140 S141 L120 L121 S142 S143 S144 S145 L63 | L63 S145 S146 L122 L123 L118 L119 S136 S137 | S226 S227 S228 L63 S234 S235 S236 S237 S230 | L63 S231 S232 S233 S234 S228 S229 | S172 S173 S174 S175 S176 L130 L131 S177 S178 S179 S180 L63 | L63 S180 S181 L132 L133 L128 L129 S171 S172 | S191 L136 L63 | L151 L152 S223 S224 S225 S207 S208 L145 L146 S209 S210 S211 S212 L147 S213 L63 | L63 S213 S214 S215 S216 S217 L148 L149 S218 S219 S220 S221 S222 L150 L151 | L64 L65 L66 L67 | L68 L69 L70 L71 | L79 L80 L81 L82 | L93 L94 L95 L96 | L114 L115 L116 L117 | L124 L125 L126 L127 | L141 L142 L143 L144
thicken "Thicken1" operation cut thickness 0.05 both sides no extend neighbours no toward (0.1604113, -0.9870503, 0) faces at (15.401, 7.5324, 6.6667)
thicken "Thicken2" operation cut thickness 0.1 both sides no extend neighbours no toward (0.1604113, -0.9870503, 0) faces at (25.401, 7.5324, 6.6667)
thicken "Thicken3" operation cut thickness 0.15 both sides no extend neighbours no toward (0.1604113, -0.9870503, 0) faces at (35.401, 7.5324, 6.6667)
thicken "Thicken4" operation cut thickness 0.2 both sides no extend neighbours no toward (0.1604113, -0.9870503, 0) faces at (45.401, 7.5324, 6.6667)
thicken "Thicken5" operation cut thickness 0.25 both sides no extend neighbours no toward (0.1604113, -0.9870503, 0) faces at (55.401, 7.5324, 6.6667)
thicken "Thicken6" operation cut thickness 0.3 both sides no extend neighbours no toward (0.1604113, -0.9870503, 0) faces at (65.401, 7.5324, 6.6667)
body "Solid1"
